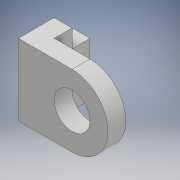
# Autodesk Inventor part: 35
Saved by Autodesk Inventor 2017 (Build 210142000, 142)
## iProperties
Part Number: 35
Material: 一般
Document SubType Name: Modeling
Designer: Brian
Density: 1 g/cm^3
Appearance: 預設
Author: Brian
Autodesk Inventor part; units mm, degrees
ref_plane "YZ Plane" through (0, 0, 0) normal (1, 0, 0) x (0, 1, 0)
ref_plane "XZ Plane" through (0, 0, 0) normal (0, 1, 0) x (-1, 0, 0)
ref_plane "XY Plane" through (0, 0, 0) normal (0, 0, 1) x (1, 0, 0)
sketch "草圖1" plane through (0, 0, 0) normal (0, 1, 0) x (-1, 0, 0)
  line L0 (0, 0) -> (-50, 0)
  line L1 (-50, 0) -> (-50, -40)
  line L2 (-50, -40) -> (0, -40)
  line L3 (0, -40) -> (0, 0)
  dimension "d0" = 50
  dimension "d1" = 40
  constraints: 8 end point, 2 parallel, 1 horizontal, 1 perpendicular
  measures "d0" distance of L1.end L2.end
  measures "d1" distance of L0.end L1.end
extrude "擠出1" add sketch "草圖1" along normal blind 10
sketch "草圖2" plane through (0, 0, -40) normal (-1, 0, 0) x (0, 0, 1)
  line L0 (0, 0) -> (0, 10) projected
  line L1 (0, 10) -> (40, 10)
  line L2 (40, 10) -> (40, 20)
  line L3 (40, 20) -> (0, 20)
  line L4 (0, 20) -> (0, 10)
  line L5 (0, 20) -> (30, 20)
  line L6 (30, 20) -> (30, 30)
  line L7 (30, 30) -> (0, 30)
  line L8 (0, 30) -> (0, 20)
  point P0 (40, 0)
  dimension "d4" = 30
  dimension "d5" = 40
  dimension "d6" = 10
  dimension "d7" = 10
  constraints: 16 end point, 4 parallel, 2 horizontal, 2 perpendicular
  measures "d4" distance of L6.end L7.end
  measures "d5" distance of L2.end L3.end
  measures "d6" distance of L3.end L0.end
  measures "d7" distance of L7.end L3.end
extrude "擠出2" add sketch "草圖2" against normal blind 10
fillet "圓角1" radius 20 2 edges at (50, 5, 0) (50, 5, -40)
hole "孔1" at (30, 0, -20) direction (0, 1, 0) diameter 20 depth 10 tip angle 118
